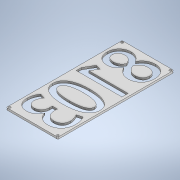
# Autodesk Inventor part: number_plate
Saved by Autodesk Inventor 2022 (Build 260153000, 153)
## iProperties
Created: 2021-07-20
Part Number: number_plate
Material: Generic
Document SubType Name: Modeling
Designer: gfellows
Density: 1 g/cm^3
Appearance: Default
Author: gfellows
Autodesk Inventor part; units mm, degrees
ref_plane "YZ Plane" through (0, 0, 0) normal (1, 0, 0) x (0, 1, 0)
ref_plane "XZ Plane" through (0, 0, 0) normal (0, 1, 0) x (-1, 0, 0)
ref_plane "XY Plane" through (0, 0, 0) normal (0, 0, 1) x (1, 0, 0)
sketch "Sketch1" plane through (0, 0, 0) normal (0, 1, 0) x (-1, 0, 0)
  line L0 (0, 0) -> (81.5, 0)
  line L1 (81.5, 0) -> (81.5, -183.1)
  line L2 (81.5, -183.1) -> (0, -183.1)
  line L3 (0, -183.1) -> (0, 0)
  line L4 (0, 0) -> (81.5, -183.1) construction
  line L5 (78.85, -2.65) -> (2.65, -2.65) construction
  line L6 (2.65, -2.65) -> (2.65, -180.45) construction
  line L7 (2.65, -180.45) -> (78.85, -180.45) construction
  line L8 (78.85, -180.45) -> (78.85, -2.65) construction
  line L9 (78.85, -2.65) -> (2.65, -180.45) construction
  line L10 (2.65, -2.65) -> (78.85, -180.45) construction
  circle A0 centre (78.85, -2.65) radius 1.65
  circle A1 centre (78.85, -180.45) radius 1.65
  circle A2 centre (2.65, -180.45) radius 1.65
  circle A3 centre (2.65, -2.65) radius 1.65
  point P0 (40.75, -91.55)
  dimension "d0" = 81.5
  dimension "d1" = 183.1
  dimension "d2" = 76.2
  dimension "d3" = 177.8
  dimension "d4" = 3.3
  dimension "d5" = 3.3
  dimension "d6" = 3.3
  dimension "d7" = 3.3
  constraints: 22 end point, 4 centre point, 4 coincident, 4 parallel, 3 midpoint, 2 horizontal, 2 perpendicular
  measures "d0" distance of L1.end L2.end
  measures "d1" distance of L2.end L0.start
  measures "d2" distance of L7.end L6.end
  measures "d3" distance of L6.end L5.end
  measures "d4" diameter of A0
  measures "d5" diameter of A1
  measures "d6" diameter of A2
  measures "d7" diameter of A3
extrude "Extrusion1" add sketch "Sketch1" along normal blind 3.175
fillet "Fillet1" radius 1.5 4 edges at (0, 1.5875, 0) (0, 1.5875, -183.1) (-81.5, 1.5875, -183.1) (-81.5, 1.5875, 0)
sketch "Sketch3" plane through (0, 0, 0) normal (0, -1, 0) x (1, 0, 0)
  arc A0 (-80, 0) -> (-81.5, -1.5) centre (-80, -1.5) ccw projected
  line L0 (-81.5, -181.6) -> (-81.5, -1.5) projected
  arc A1 (-81.5, -181.6) -> (-80, -183.1) centre (-80, -181.6) ccw projected
  line L1 (-1.5, -183.1) -> (-80, -183.1) projected
  arc A2 (-1.5, -183.1) -> (0, -181.6) centre (-1.5, -181.6) ccw projected
  line L2 (0, -1.5) -> (0, -181.6) projected
  arc A3 (0, -1.5) -> (-1.5, 0) centre (-1.5, -1.5) ccw projected
  line L3 (-80, 0) -> (-1.5, 0) projected
  circle A4 centre (-2.65, -2.65) radius 1.65 projected
  circle A5 centre (-2.65, -180.45) radius 1.65 projected
  circle A6 centre (-78.85, -180.45) radius 1.65 projected
  circle A7 centre (-78.85, -2.65) radius 1.65 projected
  circle A8 centre (-2.65, -180.45) radius 1.65 construction
  line L4 (-4.3, -180.45) -> (-4.3, -2.65) construction
  spline S0 degree 2 poles (-42.1856, -165.1433) (-39.4293, -170.4801) (-29.5766, -176.9312) (-22.6564, -177.0485) knots 0 0 0 1 2 2 2
  spline S1 degree 2 poles (-22.6564, -177.0485) (-17.4955, -177.0485) (-8.6985, -172.2981) (-3.303, -163.0906) (-3.2444, -156.4049) knots 0 0 0 1 2 3 3 3
  spline S2 degree 2 poles (-3.2444, -156.4049) (-3.303, -150.2471) (-8.5225, -140.6877) (-17.9646, -135.2335) (-24.2985, -135.1749) knots 0 0 0 1 2 3 3 3
  spline S3 degree 2 poles (-24.2985, -135.1749) (-30.9255, -135.2922) (-40.3089, -141.9193) (-42.948, -147.3147) knots 0 0 0 1 2 2 2
  line L5 (-42.948, -147.3147) -> (-43.2413, -147.3147)
  spline S4 degree 2 poles (-43.2413, -147.3147) (-46.3495, -142.0952) (-55.2638, -137.2862) (-59.9555, -137.3448) knots 0 0 0 1 2 2 2
  spline S5 degree 2 poles (-59.9555, -137.3448) (-64.4127, -137.3448) (-72.5645, -141.2741) (-77.7254, -149.3674) (-77.8427, -155.5839) knots 0 0 0 1 2 3 3 3
  spline S6 degree 2 poles (-77.8427, -155.5839) (-77.7841, -161.038) (-73.0337, -169.7177) (-64.4127, -174.7613) (-58.6067, -174.8199) knots 0 0 0 1 2 3 3 3
  spline S7 degree 2 poles (-58.6067, -174.8199) (-53.8563, -174.8199) (-45.3525, -170.0109) (-42.4789, -165.1433) knots 0 0 0 1 2 2 2
  line L6 (-42.4789, -165.1433) -> (-42.1856, -165.1433)
  spline S8 degree 2 poles (-11.103, -156.1703) (-11.2203, -161.2139) (-18.4925, -166.9027) (-24.0052, -166.9613) knots 0 0 0 1 2 2 2
  spline S9 degree 2 poles (-24.0052, -166.9613) (-28.8729, -166.9613) (-36.5556, -161.9177) (-38.4323, -157.1673) knots 0 0 0 1 2 2 2
  spline S10 degree 2 poles (-38.4323, -157.1673) (-36.4969, -151.7719) (-29.2248, -145.3207) (-23.2428, -145.2621) knots 0 0 0 1 2 2 2
  spline S11 degree 2 poles (-23.2428, -145.2621) (-18.0819, -145.2621) (-11.2203, -150.9508) (-11.103, -156.1703) knots 0 0 0 1 2 2 2
  spline S12 degree 2 poles (-70.0427, -155.9358) (-69.9841, -152.7102) (-66.8172, -148.6636) (-61.7736, -146.8456) (-58.8999, -146.8456) knots 0 0 0 1 2 3 3 3
  spline S13 degree 2 poles (-58.8999, -146.8456) (-54.5014, -146.9042) (-47.933, -151.4786) (-46.4082, -154.9388) knots 0 0 0 1 2 2 2
  spline S14 degree 2 poles (-46.4082, -154.9388) (-48.1089, -159.6305) (-54.3255, -165.2606) (-59.2518, -165.3192) knots 0 0 0 1 2 2 2
  spline S15 degree 2 poles (-59.2518, -165.3192) (-62.0668, -165.3192) (-66.9345, -163.2666) (-69.9841, -159.1027) (-70.0427, -155.9358) knots 0 0 0 1 2 3 3 3
  line L7 (-4.3, -105.7007) -> (-76.6698, -105.7007)
  line L8 (-76.6698, -105.7007) -> (-76.6698, -114.1458)
  line L9 (-76.6698, -114.1458) -> (-67.9315, -128.8074)
  line L10 (-67.9315, -128.8074) -> (-59.7209, -126.5788)
  line L11 (-59.7209, -126.5788) -> (-66.4653, -115.6119)
  line L12 (-66.4653, -115.6119) -> (-66.4653, -115.436)
  line L13 (-66.4653, -115.436) -> (-4.3, -115.436)
  line L14 (-4.3, -115.436) -> (-4.3, -105.7007)
  spline S16 degree 2 poles (-3.2444, -70.2445) (-3.303, -60.1573) (-22.6564, -49.0144) (-41.13, -48.9558) knots 0 0 0 1 2 2 2
  spline S17 degree 2 poles (-41.13, -48.9558) (-52.1555, -48.9558) (-68.6352, -53.5302) (-77.7841, -62.7377) (-77.8427, -69.5994) knots 0 0 0 1 2 3 3 3
  spline S18 degree 2 poles (-77.8427, -69.5994) (-77.7254, -79.7452) (-58.1961, -91.0053) (-40.3089, -91.064) knots 0 0 0 1 2 2 2
  spline S19 degree 2 poles (-40.3089, -91.064) (-29.1661, -91.064) (-12.5105, -86.3136) (-3.303, -77.0475) (-3.2444, -70.2445) knots 0 0 0 1 2 3 3 3
  spline S20 degree 2 poles (-12.1586, -70.0685) (-12.2759, -75.2881) (-27.1135, -80.9768) (-40.7195, -80.9768) knots 0 0 0 1 2 2 2
  spline S21 degree 2 poles (-40.7195, -80.9768) (-54.3255, -80.9181) (-68.9284, -74.9362) (-68.9871, -69.9512) knots 0 0 0 1 2 2 2
  spline S22 degree 2 poles (-68.9871, -69.9512) (-68.9284, -66.1392) (-62.0082, -61.3302) (-49.3992, -59.043) (-40.7195, -59.043) knots 0 0 0 1 2 3 3 3
  spline S23 degree 2 poles (-40.7195, -59.043) (-33.0954, -58.9843) (-20.1932, -61.037) (-12.2759, -65.9046) (-12.1586, -70.0685) knots 0 0 0 1 2 3 3 3
  spline S24 degree 2 poles (-43.4759, -22.4139) (-45.8804, -16.8425) (-54.7946, -10.9192) (-60.4247, -10.8605) knots 0 0 0 1 2 2 2
  spline S25 degree 2 poles (-60.4247, -10.8605) (-65.1164, -10.8605) (-72.9164, -14.8485) (-77.7254, -22.9417) (-77.7841, -28.9823) knots 0 0 0 1 2 3 3 3
  spline S26 degree 2 poles (-77.7841, -28.9823) (-77.7254, -34.1432) (-74.6172, -42.8229) (-72.5059, -45.3447) knots 0 0 0 1 2 2 2
  line L15 (-72.5059, -45.3447) -> (-64.53, -42.8229)
  spline S27 degree 2 poles (-64.53, -42.8229) (-66.0548, -40.8875) (-68.8111, -34.7296) (-68.8698, -31.2695) knots 0 0 0 1 2 2 2
  spline S28 degree 2 poles (-68.8698, -31.2695) (-68.7525, -26.1086) (-63.0638, -21.065) (-58.6653, -21.065) knots 0 0 0 1 2 2 2
  spline S29 degree 2 poles (-58.6653, -21.065) (-54.6773, -21.1236) (-49.4578, -25.2289) (-46.936, -31.1522) (-46.936, -34.0259) knots 0 0 0 1 2 3 3 3
  line L16 (-46.936, -34.0259) -> (-46.936, -38.2484)
  line L17 (-46.936, -38.2484) -> (-38.9601, -38.2484)
  line L18 (-38.9601, -38.2484) -> (-38.9601, -33.8499)
  spline S30 degree 2 poles (-38.9601, -33.8499) (-38.9601, -29.9206) (-36.0278, -23.2349) (-29.9872, -19.1297) (-25.2954, -19.071) knots 0 0 0 1 2 3 3 3
  spline S31 degree 2 poles (-25.2954, -19.071) (-22.0112, -19.071) (-16.0293, -21.7101) (-12.2173, -27.5161) (-12.1586, -32.0905) knots 0 0 0 1 2 3 3 3
  spline S32 degree 2 poles (-12.1586, -32.0905) (-12.2759, -36.1958) (-14.915, -43.1747) (-16.2639, -44.9928) knots 0 0 0 1 2 2 2
  line L19 (-16.2639, -44.9928) -> (-7.7601, -47.5732)
  spline S33 degree 2 poles (-7.7601, -47.5732) (-5.9421, -45.1687) (-3.303, -36.7823) (-3.2444, -31.68) knots 0 0 0 1 2 2 2
  spline S34 degree 2 poles (-3.2444, -31.68) (-3.303, -24.2906) (-9.1677, -14.0861) (-18.9616, -8.8079) (-24.9436, -8.8079) knots 0 0 0 1 2 3 3 3
  spline S35 degree 2 poles (-24.9436, -8.8079) (-30.0458, -8.8665) (-37.7285, -12.5613) (-42.4789, -18.7191) (-43.2999, -22.4139) knots 0 0 0 1 2 3 3 3
  line L20 (-43.2999, -22.4139) -> (-43.4759, -22.4139)
  point P0 (0, 0)
  constraints: 3 vertical, 2 end point, 2 horizontal alignment, 2 other
extrude "Extrusion2" cut sketch "Sketch3" against normal through all contours L6 S7 S6 S5 S4 L5 S3 S2 S1 S0 | L14 L13 L12 L11 L10 L9 L8 L7 | S19 S18 S17 S16 | L20 S35 S34 S33 L19 S32 S31 S30 L18 L17 L16 S29 S28 S27 L15 S26 S25 S24
body "Solid1"
